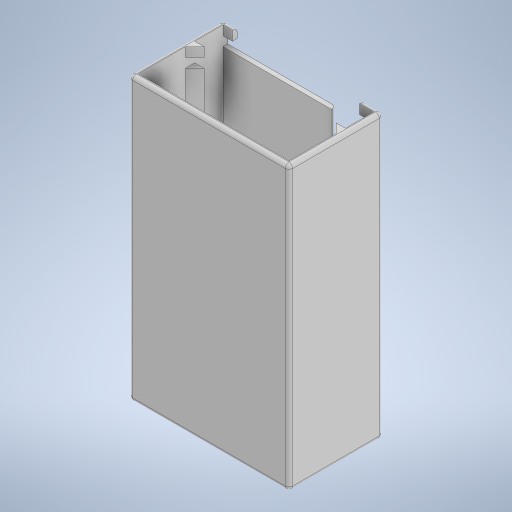
# Autodesk Inventor part: SOLDEERBOUTCASE
Saved by Autodesk Inventor 2024 (Build 280153000, 153)
## iProperties
Created: 2024-05-14
Part Number: SOLDEERBOUTCASE
Material: Generic
Document SubType Name: Modeling
Designer: Bjarni Heselmans
Density: 1 g/cm^3
Appearance: Default
Author: Bjarni Heselmans
Autodesk Inventor part; units mm, degrees
ref_plane "YZ Plane" through (0, 0, 0) normal (1, 0, 0) x (0, 1, 0)
ref_plane "XZ Plane" through (0, 0, 0) normal (0, 1, 0) x (-1, 0, 0)
ref_plane "XY Plane" through (0, 0, 0) normal (0, 0, 1) x (1, 0, 0)
sketch "Sketch1" plane through (0, 0, 0) normal (0, 0, 1) x (1, 0, 0)
  line L0 (0, 0) -> (-85, 0)
  line L1 (-85, 0) -> (-85, 50)
  line L2 (-85, 50) -> (0, 50)
  line L3 (0, 50) -> (0, 0)
  line L4 (0, 29.0147) -> (2.5, 29.0147) construction
  line L5 (-41.2407, 47.5) -> (-82.5, 47.5)
  line L6 (-82.5, 47.5) -> (-82.5, 49.429)
  line L7 (-82.5, 2.5) -> (-51.2284, 2.5)
  line L8 (-41.2407, 47.5) -> (-2.5, 47.5)
  line L9 (-2.5, 47.5) -> (-2.5, 32.5)
  line L10 (-2.5, 29.0147) -> (-2.5, 2.5)
  line L11 (-51.2284, 2.5) -> (-2.5, 2.5)
  line L12 (-82.5, 32.5) -> (-77.5, 32.5)
  line L13 (-2.5, 32.5) -> (-7.5, 32.5)
  line L14 (-77.5, 32.5) -> (-82.5, 27.5)
  line L15 (-77.5, 32.5) -> (-70.4289, 32.5) construction
  line L16 (-7.5, 32.5) -> (-2.5, 27.5)
  line L17 (-82.5, 2.5) -> (-82.5, 27.5)
  line L18 (-82.5, 32.5) -> (-82.5, 49.429)
  point P0 (-5, 32.5)
  point P1 (-80, 32.5)
  dimension "d0" = 85
  dimension "d1" = 50
  dimension "d2" = 2.5
  dimension "d10" = 5
  dimension "d11" = 5
  dimension "d12" = 135
  dimension "d27" = 2.5
  dimension "d28" = 45
  dimension "d29" = 30
  dimension "d30" = 30
  dimension "d31" = 15
  constraints: 38 end point, 6 point on line, 5 perpendicular, 4 horizontal, 2 collinear, 2 midpoint, 2 parallel, 1 equal length
  measures "d0" distance of L1.end L2.end
  measures "d1" distance of L0.end L1.end
  measures "d2" distance of L4.start L10.start
  measures "d10" distance of L12.start L12.end
  measures "d11" distance of L9.end L13.end
  measures "d12" angle of L14 L15
  measures "d27" distance between parallel lines of L0 L11
  measures "d28" distance between parallel lines of L7 L5
  measures "d29" distance from line of L11 point (-5, 32.5)
  measures "d30" distance from line of L7 point (-80, 32.5)
  measures "d31" distance from line of L5 point (-80, 32.5)
extrude "Extrusion1" add sketch "Sketch1" along normal blind 150
sketch "Sketch2" plane through (-85, 50, 0) normal (0, 1, 0) x (1, 0, 0)
  line L0 (0, 0) -> (0, -150) projected
  line L1 (85, 0) -> (85, -150) projected
  line L2 (0, 0) -> (85, 0)
  line L3 (85, 0) -> (85, -2.5)
  line L4 (85, -2.5) -> (0, -2.5)
  line L5 (0, -2.5) -> (0, 0)
  dimension "d13" = 2.5
  constraints: 8 end point, 2 parallel, 1 horizontal, 1 perpendicular, 1 point on line
  measures "d13" distance of L2.end L3.end
extrude "Extrusion2" add sketch "Sketch2" against normal blind 50
sketch "Sketch3" plane through (-85, 50, 0) normal (0, 1, 0) x (1, 0, 0)
  line L0 (0, 0) -> (85, 0) projected
  line L1 (13.6185, 0) -> (13.6185, -5)
  line L2 (13.6185, 0) -> (18.6185, 0) construction
  line L3 (0, 0) -> (0, -150) projected
  line L4 (0, -7.9354) -> (5, -7.9354)
  line L5 (0, -7.9354) -> (5, -7.9354) construction
  line L6 (2.5, -2.5) -> (2.5, -140) projected
  line L7 (5, -7.9354) -> (5, -5)
  line L8 (5, -5) -> (13.6185, -5)
  line L9 (85, 0) -> (85, -150) projected
  line L10 (85, -5) -> (80, -5)
  line L11 (85, -5) -> (90, -5) construction
  line L12 (80, -5) -> (13.6185, -5)
  line L13 (82.5, -2.5) -> (82.5, -150) projected
  line L14 (80, -5) -> (5, -5)
  line L15 (5, -5) -> (5, -35)
  line L16 (5, -35) -> (80, -35)
  line L17 (80, -35) -> (80, -5)
  dimension "d16" = 5
  dimension "d17" = 270
  dimension "d18" = 5
  dimension "d19" = 0
  dimension "d20" = 5
  dimension "d21" = 180
  dimension "d23" = 75
  dimension "d24" = 30
  constraints: 26 end point, 5 perpendicular, 4 horizontal, 4 point on line, 3 equal length, 2 parallel, 1 collinear, 1 vertical, 1 other
  measures "d16" distance of L1.start L1.end
  measures "d18" distance of L4.start L4.end
  measures "d19" distance between parallel lines of L4 L5
  measures "d20" distance of L10.start L10.end
  measures "d21" angle of L10 L11
  measures "d23" distance of L16.end L15.end
  measures "d24" distance of L15.end L14.end
extrude "Extrusion3" cut sketch "Sketch3" against normal blind 5 contours L12 L17 L16 L15 L7 L8
sketch "Sketch5" plane through (-85, 50, 0) normal (0, 1, 0) x (1, 0, 0)
  line L0 (2.5, -150) -> (82.5, -150) projected
  line L1 (13.6081, -150) -> (13.6081, -145)
  line L2 (13.6081, -145) -> (82.5, -145)
  line L3 (77.5, -2.5) -> (77.5, -150) projected
  line L4 (82.5, -145) -> (82.5, -140)
  line L5 (82.5, -140) -> (2.5, -140)
  line L6 (2.5, -140) -> (2.5, -145)
  line L7 (2.5, -145) -> (82.5, -145)
  line L8 (82.5, -145) -> (82.5, -140)
  line L9 (85, 0) -> (85, -150) projected
  line L10 (0, 0) -> (0, -150) projected
  point P0 (77.5, -145)
  point P1 (77.5, -140)
  dimension "d32" = 5
  dimension "d33" = 5
  dimension "d34" = 2.5
  dimension "d35" = 2.5
  dimension "d36" = 80
  constraints: 14 end point, 4 perpendicular, 2 parallel, 1 horizontal, 1 point on line
  measures "d32" distance of L1.start L1.end
  measures "d33" distance of L2.end L4.end
  measures "d34" distance between parallel lines of L9 L4
  measures "d35" distance between parallel lines of L10 L6
  measures "d36" distance between parallel lines of L6 L4
extrude "Extrusion4" cut sketch "Sketch5" against normal blind 47.5 contours L7 L6 L5 L3 L2 | L3 L5 L4 L2
sketch "Sketch6" plane through (-85, 50, 0) normal (0, 1, 0) x (1, 0, 0)
  line L0 (5, -35) -> (80, -35) projected
  line L1 (80, -35) -> (70, -35)
  line L2 (80, -35) -> (90, -35) construction
  line L3 (60, -45) -> (60, -35)
  line L4 (75, -45) -> (75, -35)
  line L5 (75, -150) -> (75, -45)
  line L6 (77.5, -2.5) -> (77.5, -140) projected
  line L7 (2.5, -2.5) -> (2.5, -150) projected
  line L8 (2.5, -144.4933) -> (2.5, -139.4933)
  line L9 (2.5, -139.4933) -> (7.5, -139.4933)
  line L10 (2.5, -140) -> (82.5, -140) projected
  line L11 (75, -150) -> (7.5, -150)
  line L12 (7.5, -150) -> (7.5, -139.4933)
  line L13 (7.5, -139.4933) -> (60, -139.4933)
  line L14 (75, -139.4933) -> (75, -150)
  line L15 (60, -45) -> (60, -140)
  point P0 (85, 0)
  point P1 (7.5, -140)
  dimension "d39" = 10
  dimension "d40" = 180
  dimension "d44" = 15
  dimension "d45" = 10
  dimension "d48" = 5
  dimension "d49" = 5
  dimension "d50" = 90
  constraints: 24 end point, 5 point on line, 4 parallel, 2 collinear, 2 horizontal, 2 perpendicular, 1 midpoint, 1 vertical
  measures "d39" distance of L0.end L1.end
  measures "d40" angle of L1 L2
  measures "d44" distance between parallel lines of L4 L3
  measures "d45" distance from line of L1.end L3
  measures "d48" distance of L8.start L8.end
  measures "d49" distance of L8.end L9.end
  measures "d50" angle of L8 L9
extrude "Extrusion5" cut sketch "Sketch6" against normal blind 47.5 contours L0 L4 L5 L10 L15 L3 | L10 L5 L11 L12
fillet "Fillet1" radius 2 4 edges at (-42.5, 0, 0) (0, 0, 75) (-85, 0, 75) (-42.5, 0, 150)
fillet "Fillet2" radius 2 8 edges at (-84.4142, 0.5858, 0.5858) (-85, 26, 0) (-84.4142, 0.5858, 149.4142) (-85, 26, 150) (-0.5858, 0.5858, 0.5858) (0, 26, 0) (-0.5858, 0.5858, 149.4142) (0, 26, 150)
fillet "Fillet3" radius 2 5 edges at (-52.5, 50, 35) (-42.5, 50, 5) (-5, 50, 20) (-7.5, 50, 35) (-80, 50, 20)
fillet "Fillet4" radius 2 6 edges at (-25, 49.4142, 35.5858) (-25, 47.75, 35) (-25, 50, 88.5) (-10, 49.4142, 35.5858) (-10, 47.75, 35) (-10, 50, 88.5)
fillet "Fillet5" radius 2 9 edges at (-84.4142, 50, 149.4142) (-80.25, 50, 150) (-84.4142, 50, 0.5858) (-42.5, 50, 0) (-0.5858, 50, 0.5858) (0, 50, 75) (-0.5858, 50, 149.4142) (-6, 50, 150) (-85, 50, 75)
body "Solid1"
